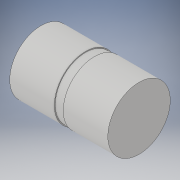
# Autodesk Inventor part: CAM_demo
Saved by Autodesk Inventor 2019 (Build 230136000, 136)
## iProperties
Created: 2021-05-16
Part Number: CAM_demo
Material: Generic
Document SubType Name: Modeling
Designer: Mike
Density: 1 g/cm^3
Appearance: Default
Author: Mike
Autodesk Inventor part; units mm, degrees
ref_plane "YZ Plane" through (0, 0, 0) normal (1, 0, 0) x (0, 1, 0)
ref_plane "XZ Plane" through (0, 0, 0) normal (0, 1, 0) x (-1, 0, 0)
ref_plane "XY Plane" through (0, 0, 0) normal (0, 0, 1) x (1, 0, 0)
sketch "Sketch1" plane through (0, 0, 0) normal (0, 0, 1) x (1, 0, 0)
  line L0 (0, 2.5) -> (0, 35)
  line L1 (0, 35) -> (50, 35)
  line L2 (50, 35) -> (50, 34)
  line L3 (50, 34) -> (60, 34)
  line L4 (60, 34) -> (60, 35)
  line L5 (60, 35) -> (110, 35)
  line L6 (110, 35) -> (110, 0)
  line L7 (110, 0) -> (30, 0)
  line L8 (0, 2.5) -> (30, 2.5)
  line L9 (30, 2.5) -> (30, 0)
  point P0 (0, 0)
  dimension "d1" = 1
  dimension "d2" = 10
  dimension "d3" = 50
  dimension "d4" = 50
  dimension "d5" = 1
  dimension "d8" = 2.5
  dimension "d9" = 35
  dimension "d10" = 30
  dimension "d12" = 30
  dimension "d14" = 110
  constraints: 20 end point, 7 perpendicular, 2 vertical, 1 horizontal
  measures "d1" distance of L1.end L2.end
  measures "d2" distance of L2.end L3.end
  measures "d3" distance of L1.end L0.end
  measures "d4" distance of L4.end L5.end
  measures "d5" distance between parallel lines of L5 L3
  measures "d8" distance from line of L8 point (0, 0)
  measures "d9" distance from line of L1 point (0, 0)
  measures "d10" distance of L7.end point (0, 0)
  measures "d12" distance from line of L9 point (0, 0)
  measures "d14" distance of L6.end point (0, 0)
revolve "Revolution1" add sketch "Sketch1" angle 360 about axis through (110, 0, 0) along (-1, 0, 0)
body "Solid1"
